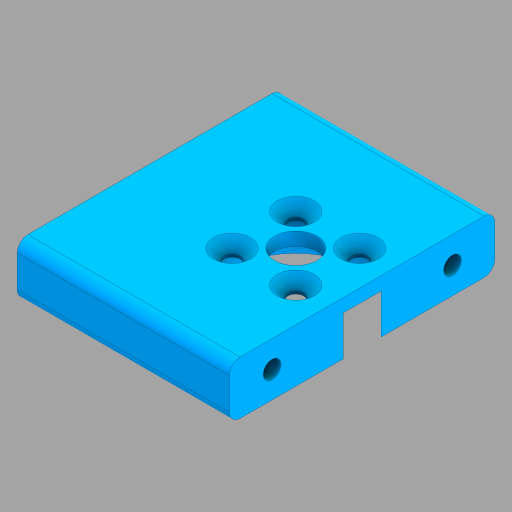
# Autodesk Inventor part: motoramma
Saved by Autodesk Inventor 2024.2 (Build 282272000, 272)
## iProperties
Created: 2023-12-16
Part Number: motoramma
Material: Типовые
Document SubType Name: Modeling
Designer: Фёдор
Density: 1 g/cm^3
Appearance: По умолчанию
Author: Фёдор
Autodesk Inventor part; units mm, degrees
ref_plane "YZ Plane" through (0, 0, 0) normal (1, 0, 0) x (0, 1, 0)
ref_plane "XZ Plane" through (0, 0, 0) normal (0, 1, 0) x (-1, 0, 0)
ref_plane "XY Plane" through (0, 0, 0) normal (0, 0, 1) x (1, 0, 0)
sketch "Эскиз1" plane through (0, 0, 0) normal (0, 1, 0) x (-1, 0, 0)
  circle A0 centre (0, 0) radius 12.5 construction
  circle A1 centre (0, 0) radius 8.5 construction
  circle A2 centre (6.0104, 6.0104) radius 1.5
  circle A3 centre (-6.0104, -6.0104) radius 1.5
  circle A4 centre (0, 0) radius 4
  line L0 (27.5, 25) -> (-12.5, 25)
  line L1 (-12.5, 25) -> (-12.5, -25)
  line L2 (-12.5, -25) -> (27.5, -25)
  line L3 (27.5, -25) -> (27.5, 25)
  line L4 (8.8388, -8.8388) -> (-8.8388, 8.8388) construction
  line L5 (-8.8388, -8.8388) -> (8.8388, 8.8388) construction
  circle A5 centre (6.0104, -6.0104) radius 1.5
  circle A6 centre (-6.0104, 6.0104) radius 1.5
  point P0 (7.5, 25)
  point P1 (7.5, -25)
  dimension "d0" = 25
  dimension "d1" = 17
  dimension "d2" = 3
  dimension "d3" = 3
  dimension "d4" = 8
  dimension "d5" = 40
  dimension "d6" = 50
  dimension "d7" = 25
  dimension "d26" = 25
  dimension "d31" = 45
  dimension "d32" = 90
  dimension "d33" = 3
  dimension "d34" = 3
  constraints: 12 end point, 8 point on circle, 7 centre point, 6 midpoint, 4 point on line, 3 coincident, 2 parallel, 1 horizontal, 1 perpendicular, 1 tangent
  measures "d0" diameter of A0
  measures "d1" diameter of A1
  measures "d2" diameter of A2
  measures "d3" diameter of A3
  measures "d4" diameter of A4
  measures "d5" distance between parallel lines of L1 L3
  measures "d6" distance of L2.end L0.start
  measures "d7" vertical distance of point (7.5, 25) point (0, 0)
  measures "d26" vertical distance of point (7.5, -25) point (0, 0)
  measures "d31" angle of L3 L5
  measures "d32" angle of L5 L4
  measures "d33" diameter of A5
  measures "d34" diameter of A6
extrude "Выдавливание1" add sketch "Эскиз1" along normal blind 2.5
sketch "Эскиз2" plane through (0, 0, 0) normal (0, -1, 0) x (1, 0, 0)
  circle A0 centre (0, 0) radius 13
  line L0 (12.5, 25) -> (12.5, -25) projected
  line L1 (-27.5, 25) -> (12.5, 25) projected
  line L2 (-27.5, -25) -> (-27.5, 25) projected
  line L3 (12.5, -25) -> (-27.5, -25) projected
  circle A1 centre (-6.0104, 6.0104) radius 1.5 projected
  circle A2 centre (6.0104, -6.0104) radius 1.5 projected
  circle A3 centre (0, 0) radius 4 projected
  point P0 (12.5, -3.5707)
  point P1 (12.5, 3.5707)
  dimension "d10" = 26
  constraints: 1 centre point, 1 coincident
  measures "d10" diameter of A0
extrude "Выдавливание2" add sketch "Эскиз2" along normal blind 7.5 contours A0 L0 L3 L2 L1
fillet "Сопряжение1" radius 2 4 edges at (-7.5, -7.5, -25) (-7.5, 2.5, -25) (-7.5, -7.5, 25) (-7.5, 2.5, 25)
sketch "Эскиз4" plane through (-27.5, -5.5, -25) normal (-1, 0, 0) x (0, 0, 1)
  arc A0 (50, 6) -> (48, 8) centre (48, 6) ccw projected
  line L0 (2, 8) -> (48, 8) projected
  arc A1 (2, 8) -> (0, 6) centre (2, 6) ccw projected
  line L1 (0, 0) -> (0, 6) projected
  arc A2 (0, 0) -> (2, -2) centre (2, 0) ccw projected
  line L2 (48, -2) -> (2, -2) projected
  arc A3 (48, -2) -> (50, 0) centre (48, 0) ccw projected
  line L3 (50, 0) -> (50, 6) projected
  circle A4 centre (42, 3) radius 1.65
  circle A5 centre (8, 3) radius 1.65
  point P0 (25, 5.5)
  point P1 (50, 3)
  dimension "d21" = 3.3
  dimension "d22" = 3.3
  dimension "d41" = 5
  dimension "d42" = 34
  dimension "d43" = 8
  dimension "d44" = 5
  constraints: 2 centre point, 1 midpoint
  measures "d21" diameter of A4
  measures "d22" diameter of A5
  measures "d41" distance from line of L2 A4.centre
  measures "d42" distance of A4.centre A5.centre
  measures "d43" distance of point (50, 3) A4.centre
  measures "d44" distance from line of L2 A5.centre
extrude "Выдавливание4" cut sketch "Эскиз4" against normal through all contours A4 | A5
chamfer "Фаска1" distance 2 angle 45 4 edges at (-4.5104, 2.5, 6.0104) (7.5104, 2.5, -6.0104) (-4.5104, 2.5, -6.0104) (7.5104, 2.5, 6.0104)
sketch "Эскиз5" plane through (0, -7.5, 0) normal (0, -1, 0) x (1, 0, 0)
  line L0 (-27.5, 23) -> (12.5, 23) projected
  line L1 (-27.5, 23) -> (-27.5, -23) projected
  line L2 (12.5, -23) -> (-27.5, -23) projected
  line L3 (12.5, -23) -> (12.5, -3.5707) projected
  arc A0 (12.5, 3.5707) -> (12.5, -3.5707) centre (0, 0) ccw projected
  line L4 (12.5, 3.5707) -> (12.5, 23) projected
  line L5 (-27.5, -18.65) -> (12.5, -18.65) projected
  line L6 (-27.5, -15.35) -> (12.5, -15.35) projected
  line L7 (12.5, -18.65) -> (12.5, -15.35)
  line L8 (12.5, -17) -> (-27.5, -17) construction
  line L9 (9, -14.1) -> (6, -14.1)
  line L10 (6, -14.1) -> (6, -19.9)
  line L11 (6, -19.9) -> (9, -19.9)
  line L12 (9, -19.9) -> (9, -14.1)
  line L13 (9, -14.1) -> (6, -19.9) construction
  line L14 (6, -14.1) -> (9, -19.9) construction
  circle A1 centre (0, 0) radius 4 projected
  line L15 (0, 0) -> (12.5, 0) construction
  line L16 (12.5, 3.5707) -> (12.5, -3.5707) projected
  line L17 (-7.5, -23) -> (-7.5, 23) construction
  line L18 (9, 14.1) -> (6, 14.1)
  line L19 (6, 14.1) -> (6, 19.9)
  line L20 (6, 19.9) -> (9, 19.9)
  line L21 (9, 19.9) -> (9, 14.1)
  line L22 (9, 14.1) -> (6, 19.9) construction
  line L23 (6, 14.1) -> (9, 19.9) construction
  line L24 (-24, -14.1) -> (-21, -14.1)
  line L25 (-21, -14.1) -> (-21, -19.9)
  line L26 (-21, -19.9) -> (-24, -19.9)
  line L27 (-24, -19.9) -> (-24, -14.1)
  line L28 (-24, -14.1) -> (-21, -19.9) construction
  line L29 (-21, -14.1) -> (-24, -19.9) construction
  line L30 (-21, 14.1) -> (-21, 19.9)
  line L31 (-21, 19.9) -> (-24, 19.9)
  line L32 (-24, 14.1) -> (-21, 14.1)
  line L33 (-24, 19.9) -> (-24, 14.1)
  line L34 (-24, 14.1) -> (-21, 19.9) construction
  line L35 (-21, 14.1) -> (-24, 19.9) construction
  point P0 (7.5, -17)
  point P1 (12.5, -13.2854)
  point P2 (7.5, 17)
  point P3 (-22.5, -17)
  point P4 (-22.5, 17)
  dimension "d35" = 3
  dimension "d36" = 5.8
  dimension "d38" = 5
  constraints: 56 end point, 15 symmetric about line, 7 midpoint, 3 perpendicular, 2 parallel, 2 point on line, 1 horizontal
  measures "d35" distance of L11.end L10.end
  measures "d36" distance of L10.end L9.end
  measures "d38" distance from line of L3 point (7.5, -17)
extrude "Выдавливание5" cut sketch "Эскиз5" against normal blind 8.5 contours L27 L24 L25 L6 | L6 L25 L5 L27 | L5 L25 L26 L27 | L10 L9 L12 L6 | L6 L12 L5 L10 | L5 L12 L11 L10 | L18 L19 L20 L21 | L32 L33 L31 L30
equation "\"d7\" = 0.5 * d6"
equation "\"d22\" = d21"
